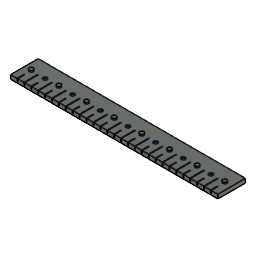
Ruler (Autodesk Fusion 360 design; units mm, degrees)
Autodesk Fusion 360 part; units mm, degrees
note: some values were not read from the file. Set by a fixed rule: which face or edge a step refers to.
sketch "Sketch1" plane through (0, 0, 0) normal (0, 0, 1) x (1, 0, 0)
  line L0 (0, 0) -> (-150, 0)
  line L1 (-150, 0) -> (-150, 20)
  line L2 (-150, 20) -> (0, 20)
  line L3 (0, 20) -> (0, 0)
  dimension "d1" = 150
  dimension "d2" = 20
  constraint horizontal L0
  constraint vertical L1
  constraint horizontal L2
  constraint vertical L3
  constraint coincident L0.start L3.end
  measures "d1" distance of L0.start L0.end
  measures "d2" distance of L0.start L2.end
extrude "Extrude1" add sketch "Sketch1" along normal blind 3
sketch "Sketch2" plane through (0, 0, 3) normal (0, 0, 1) x (-1, 0, 0)
  line L0 (0, -20) -> (150, -20)
  line L1 (150, -20) -> (150, 0)
  line L2 (150, 0) -> (0, 0)
  line L3 (0, 0) -> (0, -20)
  line L4 (150, 0) -> (145, 0)
  line L5 (145, 0) -> (145.2, 0)
  line L6 (145.2, 0) -> (145.2, -5)
  line L7 (145.2, -5) -> (145, -5)
  line L8 (145, -5) -> (145, 0)
  line L9 (145, 0) -> (144.8, 0)
  line L10 (144.8, 0) -> (144.8, -5)
  line L11 (144.8, -5) -> (145, -5)
  line L12 (145, -5) -> (145, 0)
  dimension "d5" = 0.2
  dimension "d6" = 5
  dimension "d7" = 5
  constraint coincident L1.end L2.start
  constraint coincident L2 L4.end
  constraint horizontal L5
  constraint vertical L6
  constraint horizontal L7
  constraint vertical L8
  constraint horizontal L9
  constraint vertical L10
  constraint horizontal L11
  constraint vertical L12
  measures "d5" distance of L4.end L5.end
  measures "d6" distance of L4.end L7.end
  measures "d7" distance of L4.end L7.end
extrude "Extrude2" cut sketch "Sketch2" against normal blind 2 contours L2 L8 L9 L10 L11 L12 | L2 L4 L5 L6 L7 L8 L12
pattern_linear "R-Pattern1" count 29 spacing 5 along (1, 0, 0) of "Extrude2"
extrude "Extrude3" cut 14 faces at (-139.9333, 5, 2.3333) (-129.9333, 5, 2.3333) (-119.9333, 5, 2.3333) (-109.9333, 5, 2.3333) (-99.9333, 5, 2.3333) (-89.9333, 5, 2.3333) (-79.9333, 5, 2.3333) (-69.9333, 5, 2.3333) (-59.9333, 5, 2.3333) (-49.9333, 5, 2.3333) (-39.9333, 5, 2.3333) (-29.9333, 5, 2.3333) (-19.9333, 5, 2.3333) (-9.9333, 5, 2.3333) along direction (0, 1, 0) blind 5
sketch "Sketch3" plane through (0, 0, 3) normal (0, 0, 1) x (-1, 0, 0)
  line L0 (19.8, -10) -> (19.8, 0)
  line L1 (19.8, 0) -> (15.2, 0)
  line L2 (15.2, 0) -> (15.2, -5)
  line L3 (15.2, -5) -> (14.8, -5)
  line L4 (14.8, -5) -> (14.8, 0)
  line L5 (14.8, 0) -> (10.2, 0)
  line L6 (10.2, 0) -> (10.2, -10)
  line L7 (10.2, -10) -> (9.8, -10)
  line L8 (9.8, -10) -> (9.8, 0)
  line L9 (9.8, 0) -> (5.2, 0)
  line L10 (5.2, 0) -> (5.2, -5)
  line L11 (5.2, -5) -> (4.8, -5)
  line L12 (4.8, -5) -> (4.8, 0)
  line L13 (4.8, 0) -> (0, 0)
  line L14 (0, 0) -> (0, -20)
  line L15 (0, -20) -> (150, -20)
  line L16 (150, -20) -> (150, 0)
  line L17 (150, 0) -> (145.2, 0)
  line L18 (145.2, 0) -> (145.2, -5)
  line L19 (145.2, -5) -> (144.8, -5)
  line L20 (144.8, -5) -> (144.8, 0)
  line L21 (144.8, 0) -> (140.2, 0)
  line L22 (140.2, 0) -> (140.2, -10)
  line L23 (140.2, -10) -> (139.8, -10)
  line L24 (139.8, -10) -> (139.8, 0)
  line L25 (139.8, 0) -> (135.2, 0)
  line L26 (135.2, 0) -> (135.2, -5)
  line L27 (135.2, -5) -> (134.8, -5)
  line L28 (134.8, -5) -> (134.8, 0)
  line L29 (134.8, 0) -> (130.2, 0)
  line L30 (130.2, 0) -> (130.2, -10)
  line L31 (130.2, -10) -> (129.8, -10)
  line L32 (129.8, -10) -> (129.8, 0)
  line L33 (129.8, 0) -> (125.2, 0)
  line L34 (125.2, 0) -> (125.2, -5)
  line L35 (125.2, -5) -> (124.8, -5)
  line L36 (124.8, -5) -> (124.8, 0)
  line L37 (124.8, 0) -> (120.2, 0)
  line L38 (120.2, 0) -> (120.2, -10)
  line L39 (120.2, -10) -> (119.8, -10)
  line L40 (119.8, -10) -> (119.8, 0)
  line L41 (119.8, 0) -> (115.2, 0)
  line L42 (115.2, 0) -> (115.2, -5)
  line L43 (115.2, -5) -> (114.8, -5)
  line L44 (114.8, -5) -> (114.8, 0)
  line L45 (114.8, 0) -> (110.2, 0)
  line L46 (110.2, 0) -> (110.2, -10)
  line L47 (110.2, -10) -> (109.8, -10)
  line L48 (109.8, -10) -> (109.8, 0)
  line L49 (109.8, 0) -> (105.2, 0)
  line L50 (105.2, 0) -> (105.2, -5)
  line L51 (105.2, -5) -> (104.8, -5)
  line L52 (104.8, -5) -> (104.8, 0)
  line L53 (104.8, 0) -> (100.2, 0)
  line L54 (100.2, 0) -> (100.2, -10)
  line L55 (100.2, -10) -> (99.8, -10)
  line L56 (99.8, -10) -> (99.8, 0)
  line L57 (99.8, 0) -> (95.2, 0)
  line L58 (95.2, 0) -> (95.2, -5)
  line L59 (95.2, -5) -> (94.8, -5)
  line L60 (94.8, -5) -> (94.8, 0)
  line L61 (94.8, 0) -> (90.2, 0)
  line L62 (90.2, 0) -> (90.2, -10)
  line L63 (90.2, -10) -> (89.8, -10)
  line L64 (89.8, -10) -> (89.8, 0)
  line L65 (89.8, 0) -> (85.2, 0)
  line L66 (85.2, 0) -> (85.2, -5)
  line L67 (85.2, -5) -> (84.8, -5)
  line L68 (84.8, -5) -> (84.8, 0)
  line L69 (84.8, 0) -> (80.2, 0)
  line L70 (80.2, 0) -> (80.2, -10)
  line L71 (80.2, -10) -> (79.8, -10)
  line L72 (79.8, -10) -> (79.8, 0)
  line L73 (79.8, 0) -> (75.2, 0)
  line L74 (75.2, 0) -> (75.2, -5)
  line L75 (75.2, -5) -> (74.8, -5)
  line L76 (74.8, -5) -> (74.8, 0)
  line L77 (74.8, 0) -> (70.2, 0)
  line L78 (70.2, 0) -> (70.2, -10)
  line L79 (70.2, -10) -> (69.8, -10)
  line L80 (69.8, -10) -> (69.8, 0)
  line L81 (69.8, 0) -> (65.2, 0)
  line L82 (65.2, 0) -> (65.2, -5)
  line L83 (65.2, -5) -> (64.8, -5)
  line L84 (64.8, -5) -> (64.8, 0)
  line L85 (64.8, 0) -> (60.2, 0)
  line L86 (60.2, 0) -> (60.2, -10)
  line L87 (60.2, -10) -> (59.8, -10)
  line L88 (59.8, -10) -> (59.8, 0)
  line L89 (59.8, 0) -> (55.2, 0)
  line L90 (55.2, 0) -> (55.2, -5)
  line L91 (55.2, -5) -> (54.8, -5)
  line L92 (54.8, -5) -> (54.8, 0)
  line L93 (54.8, 0) -> (50.2, 0)
  line L94 (50.2, 0) -> (50.2, -10)
  line L95 (50.2, -10) -> (49.8, -10)
  line L96 (49.8, -10) -> (49.8, 0)
  line L97 (49.8, 0) -> (45.2, 0)
  line L98 (45.2, 0) -> (45.2, -5)
  line L99 (45.2, -5) -> (44.8, -5)
  line L100 (44.8, -5) -> (44.8, 0)
  line L101 (44.8, 0) -> (40.2, 0)
  line L102 (40.2, 0) -> (40.2, -10)
  line L103 (40.2, -10) -> (39.8, -10)
  line L104 (39.8, -10) -> (39.8, 0)
  line L105 (39.8, 0) -> (35.2, 0)
  line L106 (35.2, 0) -> (35.2, -5)
  line L107 (35.2, -5) -> (34.8, -5)
  line L108 (34.8, -5) -> (34.8, 0)
  line L109 (34.8, 0) -> (30.2, 0)
  line L110 (30.2, 0) -> (30.2, -10)
  line L111 (30.2, -10) -> (29.8, -10)
  line L112 (29.8, -10) -> (29.8, 0)
  line L113 (29.8, 0) -> (25.2, 0)
  line L114 (25.2, 0) -> (25.2, -5)
  line L115 (25.2, -5) -> (24.8, -5)
  line L116 (24.8, -5) -> (24.8, 0)
  line L117 (24.8, 0) -> (20.2, 0)
  line L118 (20.2, 0) -> (20.2, -10)
  line L119 (20.2, -10) -> (19.8, -10)
  circle A0 centre (145, -10) radius 1.5
  dimension "d16" = 3
  measures "d16" diameter of A0
extrude "Extrude4" add sketch "Sketch3" along normal blind 1 contours A0
pattern_linear "R-Pattern2" count 8 spacing 20 along (1, 0, 0) of "Extrude4"
sketch "Sketch4" plane through (0, 0, 3) normal (0, 0, 1) x (-1, 0, 0)
  circle A0 centre (5, -10) radius 1.5
  circle A1 centre (25, -10) radius 1.5
  circle A2 centre (45, -10) radius 1.5
  circle A3 centre (65, -10) radius 1.5
  circle A4 centre (85, -10) radius 1.5
  circle A5 centre (105, -10) radius 1.5
  circle A6 centre (125, -10) radius 1.5
  circle A7 centre (145, -10) radius 1.5
  line L0 (19.8, -10) -> (19.8, 0)
  line L1 (19.8, 0) -> (15.2, 0)
  line L2 (15.2, 0) -> (15.2, -5)
  line L3 (15.2, -5) -> (14.8, -5)
  line L4 (14.8, -5) -> (14.8, 0)
  line L5 (14.8, 0) -> (10.2, 0)
  line L6 (10.2, 0) -> (10.2, -10)
  line L7 (10.2, -10) -> (9.8, -10)
  line L8 (9.8, -10) -> (9.8, 0)
  line L9 (9.8, 0) -> (5.2, 0)
  line L10 (5.2, 0) -> (5.2, -5)
  line L11 (5.2, -5) -> (4.8, -5)
  line L12 (4.8, -5) -> (4.8, 0)
  line L13 (4.8, 0) -> (0, 0)
  line L14 (0, 0) -> (0, -20)
  line L15 (0, -20) -> (150, -20)
  line L16 (150, -20) -> (150, 0)
  line L17 (150, 0) -> (145.2, 0)
  line L18 (145.2, 0) -> (145.2, -5)
  line L19 (145.2, -5) -> (144.8, -5)
  line L20 (144.8, -5) -> (144.8, 0)
  line L21 (144.8, 0) -> (140.2, 0)
  line L22 (140.2, 0) -> (140.2, -10)
  line L23 (140.2, -10) -> (139.8, -10)
  line L24 (139.8, -10) -> (139.8, 0)
  line L25 (139.8, 0) -> (135.2, 0)
  line L26 (135.2, 0) -> (135.2, -5)
  line L27 (135.2, -5) -> (134.8, -5)
  line L28 (134.8, -5) -> (134.8, 0)
  line L29 (134.8, 0) -> (130.2, 0)
  line L30 (130.2, 0) -> (130.2, -10)
  line L31 (130.2, -10) -> (129.8, -10)
  line L32 (129.8, -10) -> (129.8, 0)
  line L33 (129.8, 0) -> (125.2, 0)
  line L34 (125.2, 0) -> (125.2, -5)
  line L35 (125.2, -5) -> (124.8, -5)
  line L36 (124.8, -5) -> (124.8, 0)
  line L37 (124.8, 0) -> (120.2, 0)
  line L38 (120.2, 0) -> (120.2, -10)
  line L39 (120.2, -10) -> (119.8, -10)
  line L40 (119.8, -10) -> (119.8, 0)
  line L41 (119.8, 0) -> (115.2, 0)
  line L42 (115.2, 0) -> (115.2, -5)
  line L43 (115.2, -5) -> (114.8, -5)
  line L44 (114.8, -5) -> (114.8, 0)
  line L45 (114.8, 0) -> (110.2, 0)
  line L46 (110.2, 0) -> (110.2, -10)
  line L47 (110.2, -10) -> (109.8, -10)
  line L48 (109.8, -10) -> (109.8, 0)
  line L49 (109.8, 0) -> (105.2, 0)
  line L50 (105.2, 0) -> (105.2, -5)
  line L51 (105.2, -5) -> (104.8, -5)
  line L52 (104.8, -5) -> (104.8, 0)
  line L53 (104.8, 0) -> (100.2, 0)
  line L54 (100.2, 0) -> (100.2, -10)
  line L55 (100.2, -10) -> (99.8, -10)
  line L56 (99.8, -10) -> (99.8, 0)
  line L57 (99.8, 0) -> (95.2, 0)
  line L58 (95.2, 0) -> (95.2, -5)
  line L59 (95.2, -5) -> (94.8, -5)
  line L60 (94.8, -5) -> (94.8, 0)
  line L61 (94.8, 0) -> (90.2, 0)
  line L62 (90.2, 0) -> (90.2, -10)
  line L63 (90.2, -10) -> (89.8, -10)
  line L64 (89.8, -10) -> (89.8, 0)
  line L65 (89.8, 0) -> (85.2, 0)
  line L66 (85.2, 0) -> (85.2, -5)
  line L67 (85.2, -5) -> (84.8, -5)
  line L68 (84.8, -5) -> (84.8, 0)
  line L69 (84.8, 0) -> (80.2, 0)
  line L70 (80.2, 0) -> (80.2, -10)
  line L71 (80.2, -10) -> (79.8, -10)
  line L72 (79.8, -10) -> (79.8, 0)
  line L73 (79.8, 0) -> (75.2, 0)
  line L74 (75.2, 0) -> (75.2, -5)
  line L75 (75.2, -5) -> (74.8, -5)
  line L76 (74.8, -5) -> (74.8, 0)
  line L77 (74.8, 0) -> (70.2, 0)
  line L78 (70.2, 0) -> (70.2, -10)
  line L79 (70.2, -10) -> (69.8, -10)
  line L80 (69.8, -10) -> (69.8, 0)
  line L81 (69.8, 0) -> (65.2, 0)
  line L82 (65.2, 0) -> (65.2, -5)
  line L83 (65.2, -5) -> (64.8, -5)
  line L84 (64.8, -5) -> (64.8, 0)
  line L85 (64.8, 0) -> (60.2, 0)
  line L86 (60.2, 0) -> (60.2, -10)
  line L87 (60.2, -10) -> (59.8, -10)
  line L88 (59.8, -10) -> (59.8, 0)
  line L89 (59.8, 0) -> (55.2, 0)
  line L90 (55.2, 0) -> (55.2, -5)
  line L91 (55.2, -5) -> (54.8, -5)
  line L92 (54.8, -5) -> (54.8, 0)
  line L93 (54.8, 0) -> (50.2, 0)
  line L94 (50.2, 0) -> (50.2, -10)
  line L95 (50.2, -10) -> (49.8, -10)
  line L96 (49.8, -10) -> (49.8, 0)
  line L97 (49.8, 0) -> (45.2, 0)
  line L98 (45.2, 0) -> (45.2, -5)
  line L99 (45.2, -5) -> (44.8, -5)
  line L100 (44.8, -5) -> (44.8, 0)
  line L101 (44.8, 0) -> (40.2, 0)
  line L102 (40.2, 0) -> (40.2, -10)
  line L103 (40.2, -10) -> (39.8, -10)
  line L104 (39.8, -10) -> (39.8, 0)
  line L105 (39.8, 0) -> (35.2, 0)
  line L106 (35.2, 0) -> (35.2, -5)
  line L107 (35.2, -5) -> (34.8, -5)
  line L108 (34.8, -5) -> (34.8, 0)
  line L109 (34.8, 0) -> (30.2, 0)
  line L110 (30.2, 0) -> (30.2, -10)
  line L111 (30.2, -10) -> (29.8, -10)
  line L112 (29.8, -10) -> (29.8, 0)
  line L113 (29.8, 0) -> (25.2, 0)
  line L114 (25.2, 0) -> (25.2, -5)
  line L115 (25.2, -5) -> (24.8, -5)
  line L116 (24.8, -5) -> (24.8, 0)
  line L117 (24.8, 0) -> (20.2, 0)
  line L118 (20.2, 0) -> (20.2, -10)
  line L119 (20.2, -10) -> (19.8, -10)
  circle A8 centre (135, -10) radius 1.5
  dimension "d23" = 3
  measures "d23" diameter of A8
extrude "Extrude5" cut sketch "Sketch4" against normal blind 1 contours A8
pattern_linear "R-Pattern3" count 8 spacing 20 along (1, 0, 0) of "Extrude5"
sketch "Sketch5" plane through (0, 0, 3) normal (0, 0, 1) x (-1, 0, 0)
  circle A0 centre (15, -10) radius 1.5
  circle A1 centre (35, -10) radius 1.5
  circle A2 centre (55, -10) radius 1.5
  circle A3 centre (75, -10) radius 1.5
  circle A4 centre (95, -10) radius 1.5
  circle A5 centre (115, -10) radius 1.5
  circle A6 centre (135, -10) radius 1.5
  circle A7 centre (5, -10) radius 1.5
  circle A8 centre (25, -10) radius 1.5
  circle A9 centre (45, -10) radius 1.5
  circle A10 centre (65, -10) radius 1.5
  circle A11 centre (85, -10) radius 1.5
  circle A12 centre (105, -10) radius 1.5
  circle A13 centre (125, -10) radius 1.5
  circle A14 centre (145, -10) radius 1.5
  line L0 (19.8, -10) -> (19.8, 0)
  line L1 (19.8, 0) -> (15.2, 0)
  line L2 (15.2, 0) -> (15.2, -5)
  line L3 (15.2, -5) -> (14.8, -5)
  line L4 (14.8, -5) -> (14.8, 0)
  line L5 (14.8, 0) -> (10.2, 0)
  line L6 (10.2, 0) -> (10.2, -10)
  line L7 (10.2, -10) -> (9.8, -10)
  line L8 (9.8, -10) -> (9.8, 0)
  line L9 (9.8, 0) -> (5.2, 0)
  line L10 (5.2, 0) -> (5.2, -5)
  line L11 (5.2, -5) -> (4.8, -5)
  line L12 (4.8, -5) -> (4.8, 0)
  line L13 (4.8, 0) -> (0, 0)
  line L14 (0, 0) -> (0, -20)
  line L15 (0, -20) -> (150, -20)
  line L16 (150, -20) -> (150, 0)
  line L17 (150, 0) -> (145.2, 0)
  line L18 (145.2, 0) -> (145.2, -5)
  line L19 (145.2, -5) -> (144.8, -5)
  line L20 (144.8, -5) -> (144.8, 0)
  line L21 (144.8, 0) -> (140.2, 0)
  line L22 (140.2, 0) -> (140.2, -10)
  line L23 (140.2, -10) -> (139.8, -10)
  line L24 (139.8, -10) -> (139.8, 0)
  line L25 (139.8, 0) -> (135.2, 0)
  line L26 (135.2, 0) -> (135.2, -5)
  line L27 (135.2, -5) -> (134.8, -5)
  line L28 (134.8, -5) -> (134.8, 0)
  line L29 (134.8, 0) -> (130.2, 0)
  line L30 (130.2, 0) -> (130.2, -10)
  line L31 (130.2, -10) -> (129.8, -10)
  line L32 (129.8, -10) -> (129.8, 0)
  line L33 (129.8, 0) -> (125.2, 0)
  line L34 (125.2, 0) -> (125.2, -5)
  line L35 (125.2, -5) -> (124.8, -5)
  line L36 (124.8, -5) -> (124.8, 0)
  line L37 (124.8, 0) -> (120.2, 0)
  line L38 (120.2, 0) -> (120.2, -10)
  line L39 (120.2, -10) -> (119.8, -10)
  line L40 (119.8, -10) -> (119.8, 0)
  line L41 (119.8, 0) -> (115.2, 0)
  line L42 (115.2, 0) -> (115.2, -5)
  line L43 (115.2, -5) -> (114.8, -5)
  line L44 (114.8, -5) -> (114.8, 0)
  line L45 (114.8, 0) -> (110.2, 0)
  line L46 (110.2, 0) -> (110.2, -10)
  line L47 (110.2, -10) -> (109.8, -10)
  line L48 (109.8, -10) -> (109.8, 0)
  line L49 (109.8, 0) -> (105.2, 0)
  line L50 (105.2, 0) -> (105.2, -5)
  line L51 (105.2, -5) -> (104.8, -5)
  line L52 (104.8, -5) -> (104.8, 0)
  line L53 (104.8, 0) -> (100.2, 0)
  line L54 (100.2, 0) -> (100.2, -10)
  line L55 (100.2, -10) -> (99.8, -10)
  line L56 (99.8, -10) -> (99.8, 0)
  line L57 (99.8, 0) -> (95.2, 0)
  line L58 (95.2, 0) -> (95.2, -5)
  line L59 (95.2, -5) -> (94.8, -5)
  line L60 (94.8, -5) -> (94.8, 0)
  line L61 (94.8, 0) -> (90.2, 0)
  line L62 (90.2, 0) -> (90.2, -10)
  line L63 (90.2, -10) -> (89.8, -10)
  line L64 (89.8, -10) -> (89.8, 0)
  line L65 (89.8, 0) -> (85.2, 0)
  line L66 (85.2, 0) -> (85.2, -5)
  line L67 (85.2, -5) -> (84.8, -5)
  line L68 (84.8, -5) -> (84.8, 0)
  line L69 (84.8, 0) -> (80.2, 0)
  line L70 (80.2, 0) -> (80.2, -10)
  line L71 (80.2, -10) -> (79.8, -10)
  line L72 (79.8, -10) -> (79.8, 0)
  line L73 (79.8, 0) -> (75.2, 0)
  line L74 (75.2, 0) -> (75.2, -5)
  line L75 (75.2, -5) -> (74.8, -5)
  line L76 (74.8, -5) -> (74.8, 0)
  line L77 (74.8, 0) -> (70.2, 0)
  line L78 (70.2, 0) -> (70.2, -10)
  line L79 (70.2, -10) -> (69.8, -10)
  line L80 (69.8, -10) -> (69.8, 0)
  line L81 (69.8, 0) -> (65.2, 0)
  line L82 (65.2, 0) -> (65.2, -5)
  line L83 (65.2, -5) -> (64.8, -5)
  line L84 (64.8, -5) -> (64.8, 0)
  line L85 (64.8, 0) -> (60.2, 0)
  line L86 (60.2, 0) -> (60.2, -10)
  line L87 (60.2, -10) -> (59.8, -10)
  line L88 (59.8, -10) -> (59.8, 0)
  line L89 (59.8, 0) -> (55.2, 0)
  line L90 (55.2, 0) -> (55.2, -5)
  line L91 (55.2, -5) -> (54.8, -5)
  line L92 (54.8, -5) -> (54.8, 0)
  line L93 (54.8, 0) -> (50.2, 0)
  line L94 (50.2, 0) -> (50.2, -10)
  line L95 (50.2, -10) -> (49.8, -10)
  line L96 (49.8, -10) -> (49.8, 0)
  line L97 (49.8, 0) -> (45.2, 0)
  line L98 (45.2, 0) -> (45.2, -5)
  line L99 (45.2, -5) -> (44.8, -5)
  line L100 (44.8, -5) -> (44.8, 0)
  line L101 (44.8, 0) -> (40.2, 0)
  line L102 (40.2, 0) -> (40.2, -10)
  line L103 (40.2, -10) -> (39.8, -10)
  line L104 (39.8, -10) -> (39.8, 0)
  line L105 (39.8, 0) -> (35.2, 0)
  line L106 (35.2, 0) -> (35.2, -5)
  line L107 (35.2, -5) -> (34.8, -5)
  line L108 (34.8, -5) -> (34.8, 0)
  line L109 (34.8, 0) -> (30.2, 0)
  line L110 (30.2, 0) -> (30.2, -10)
  line L111 (30.2, -10) -> (29.8, -10)
  line L112 (29.8, -10) -> (29.8, 0)
  line L113 (29.8, 0) -> (25.2, 0)
  line L114 (25.2, 0) -> (25.2, -5)
  line L115 (25.2, -5) -> (24.8, -5)
  line L116 (24.8, -5) -> (24.8, 0)
  line L117 (24.8, 0) -> (20.2, 0)
  line L118 (20.2, 0) -> (20.2, -10)
  line L119 (20.2, -10) -> (19.8, -10)
